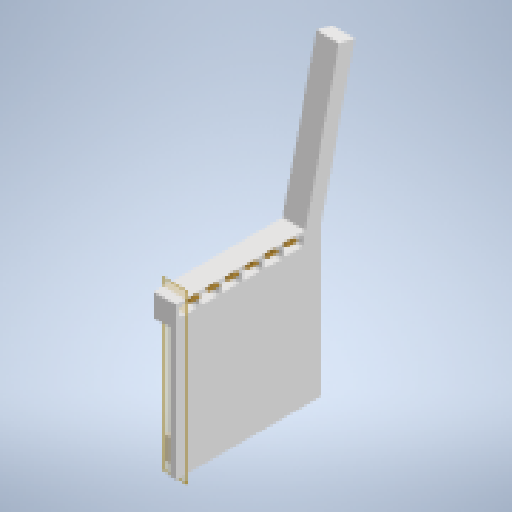
# Autodesk Inventor part: bench-end-peice
Saved by Autodesk Inventor 2023 (Build 270158030, 158C)
## iProperties
Created: 2024-09-09
Part Number: bench-end-peice
Material: Generic
Document SubType Name: Modeling
Designer: Imogen Heard
Density: 1 g/cm^3
Appearance: Default
Author: Imogen Heard
Autodesk Inventor part; units mm, degrees
ref_plane "YZ Plane" through (0, 0, 0) normal (1, 0, 0) x (0, 1, 0)
ref_plane "XZ Plane" through (0, 0, 0) normal (0, 1, 0) x (-1, 0, 0)
ref_plane "XY Plane" through (0, 0, 0) normal (0, 0, 1) x (1, 0, 0)
sketch "Sketch1" plane through (0, 0, 0) normal (1, 0, 0) x (0, 1, 0)
  line L0 (70, 190) -> (0, 190)
  line L1 (0, 190) -> (0, -190)
  line L2 (0, -190) -> (70, -190)
  line L3 (70, -190) -> (70, 190)
  line L4 (29.8496, 82.6594) -> (70, 140)
  line L5 (70, 140) -> (440.1504, -119.1821)
  line L6 (440.1504, -119.1821) -> (400, -176.5227)
  line L7 (400, -176.5227) -> (29.8496, 82.6594)
  line L8 (29.8496, 82.6594) -> (440.1504, -119.1821) construction
  line L9 (70, 140) -> (400, -176.5227) construction
  line L10 (470, 225) -> (400, 225)
  line L11 (400, 225) -> (400, -225)
  line L12 (400, -225) -> (470, -225)
  line L13 (470, -225) -> (470, 225)
  point P0 (0, 0)
  point P1 (35, 190)
  point P2 (435, -225)
  point P3 (400, -91.0685)
  point P4 (70, 54.5458)
  dimension "d0" = 380
  dimension "d1" = 70
  dimension "d2" = 190
  dimension "d3" = 70
  dimension "d4" = 50
  dimension "d5" = 400
  dimension "d6" = 55
  dimension "d7" = -13.4773
  dimension "d8" = 70
  dimension "d9" = 450
  dimension "d10" = 35
  dimension "d11" = 35
  constraints: 28 end point, 6 parallel, 3 perpendicular, 2 horizontal, 2 midpoint, 2 vertical alignment, 1 point on line
  measures "d0" distance between parallel lines of L2 L0
  measures "d1" distance between parallel lines of L3 L1
  measures "d2" distance from line of L0 point (0, 0)
  measures "d3" distance between parallel lines of L7 L5
  measures "d4" vertical distance of point (35, 190) L4.end
  measures "d5" distance from line of L6.end L1
  measures "d6" angle of L3 L7
  measures "d7" distance from line of L2 L6.end
  measures "d8" distance between parallel lines of L11 L13
  measures "d9" distance between parallel lines of L10 L12
  measures "d10" distance from line of point (435, -225) L2
  measures "d11" distance between parallel lines of L10 L0
extrude "Extrusion1" add sketch "Sketch1" along normal blind 70
sketch "Sketch2" plane through (0, 0, 0) normal (-1, 0, 0) x (0, 0, 1)
  line L0 (165, 460) -> (205, 460)
  line L1 (215, 450) -> (215, 440)
  line L2 (205, 430) -> (165, 430)
  line L3 (155, 440) -> (155, 450)
  line L4 (-225, 470) -> (225, 470) projected
  line L5 (225, 470) -> (225, 400) projected
  arc A0 (165, 460) -> (155, 450) centre (165, 450) ccw
  arc A1 (215, 450) -> (205, 460) centre (205, 450) ccw
  arc A2 (205, 430) -> (215, 440) centre (205, 440) ccw
  arc A3 (155, 440) -> (165, 430) centre (165, 440) ccw
  line L6 (100, 460) -> (140, 460)
  line L7 (150, 450) -> (150, 440)
  line L8 (140, 430) -> (100, 430)
  line L9 (90, 440) -> (90, 450)
  arc A4 (100, 460) -> (90, 450) centre (100, 450) ccw
  arc A5 (150, 450) -> (140, 460) centre (140, 450) ccw
  arc A6 (140, 430) -> (150, 440) centre (140, 440) ccw
  arc A7 (90, 440) -> (100, 430) centre (100, 440) ccw
  line L10 (35, 460) -> (75, 460)
  line L11 (85, 450) -> (85, 440)
  line L12 (75, 430) -> (35, 430)
  line L13 (25, 440) -> (25, 450)
  arc A8 (35, 460) -> (25, 450) centre (35, 450) ccw
  arc A9 (85, 450) -> (75, 460) centre (75, 450) ccw
  arc A10 (75, 430) -> (85, 440) centre (75, 440) ccw
  arc A11 (25, 440) -> (35, 430) centre (35, 440) ccw
  line L14 (-30, 460) -> (10, 460)
  line L15 (20, 450) -> (20, 440)
  line L16 (10, 430) -> (-30, 430)
  line L17 (-40, 440) -> (-40, 450)
  arc A12 (-30, 460) -> (-40, 450) centre (-30, 450) ccw
  arc A13 (20, 450) -> (10, 460) centre (10, 450) ccw
  arc A14 (10, 430) -> (20, 440) centre (10, 440) ccw
  arc A15 (-40, 440) -> (-30, 430) centre (-30, 440) ccw
  line L18 (-95, 460) -> (-55, 460)
  line L19 (-45, 450) -> (-45, 440)
  line L20 (-55, 430) -> (-95, 430)
  line L21 (-105, 440) -> (-105, 450)
  arc A16 (-95, 460) -> (-105, 450) centre (-95, 450) ccw
  arc A17 (-45, 450) -> (-55, 460) centre (-55, 450) ccw
  arc A18 (-55, 430) -> (-45, 440) centre (-55, 440) ccw
  arc A19 (-105, 440) -> (-95, 430) centre (-95, 440) ccw
  line L22 (-160, 460) -> (-120, 460)
  line L23 (-110, 450) -> (-110, 440)
  line L24 (-120, 430) -> (-160, 430)
  line L25 (-170, 440) -> (-170, 450)
  arc A20 (-160, 460) -> (-170, 450) centre (-160, 450) ccw
  arc A21 (-110, 450) -> (-120, 460) centre (-120, 450) ccw
  arc A22 (-120, 430) -> (-110, 440) centre (-120, 440) ccw
  arc A23 (-170, 440) -> (-160, 430) centre (-160, 440) ccw
  point P0 (0, 0)
  dimension "d14" = 60
  dimension "d15" = 30
  dimension "d16" = 10
  dimension "d17" = 10
  dimension "d18" = 10
  dimension "d21" = 65
  constraints: 48 end point, 48 point on circle, 24 centre point, 8 tangent, 3 equal radius, 2 horizontal, 2 parallel, 1 perpendicular, 100 other
  measures "d14" distance between parallel lines of L1 L3
  measures "d15" distance between parallel lines of L2 L0
  measures "d16" distance between parallel lines of L4 L0
  measures "d17" distance between parallel lines of L5 L1
  measures "d18" radius of A0
  measures "d21" distance of L0.start L6.start
extrude "Extrusion2" cut sketch "Sketch2" against normal through all
sketch "Sketch3" plane through (70, 0, 0) normal (1, 0, 0) x (0, 0, -1)
  line L0 (223.7185, 458.7524) -> (175, 470)
  line L1 (175, 470) -> (278.8907, 920)
  line L2 (278.8907, 920) -> (327.6092, 908.7524)
  line L3 (327.6092, 908.7524) -> (223.7185, 458.7524)
  line L4 (225, 470) -> (-225, 470) projected
  line L5 (225, 400) -> (225, 470) projected
  line L6 (-225, 470) -> (-225, 400) projected
  point P0 (0, 0)
  point P1 (-225, 435)
  point P2 (225, 435)
  dimension "d28" = 103
  dimension "d29" = 50
  dimension "d30" = 50
  dimension "d31" = 450
  dimension "d32" = 450
  constraints: 8 end point, 2 midpoint, 2 parallel, 1 perpendicular, 1 point on line
  measures "d28" angle of L1 L4
  measures "d29" distance between parallel lines of L3 L1
  measures "d30" distance from line of L5 L0.end
  measures "d31" distance from line of L1.end L4
  measures "d32" distance of point (-225, 435) point (225, 435)
extrude "Extrusion3" add sketch "Sketch3" against normal up to surface (70 mm away)
sketch "Sketch4" plane through (70, 0, 0) normal (1, 0, 0) x (0, 0, -1)
  line L0 (175, 470) -> (-225, 470) projected
  line L1 (-225, 470) -> (-225, 400) projected
  line L2 (-225, 400) -> (91.0685, 400) projected
  line L3 (91.0685, 400) -> (-140, 70) projected
  line L4 (-140, 70) -> (-190, 70) projected
  line L5 (-190, 70) -> (-190, 0) projected
  line L6 (-190, 0) -> (190, 0) projected
  line L7 (190, 0) -> (190, 70) projected
  line L8 (190, 70) -> (-54.5458, 70) projected
  line L9 (-54.5458, 70) -> (176.5227, 400) projected
  line L10 (176.5227, 400) -> (225, 400) projected
  line L11 (225, 400) -> (225, 464.3032) projected
  line L12 (225, 464.3032) -> (327.6092, 908.7524) projected
  line L13 (327.6092, 908.7524) -> (278.8907, 920) projected
  line L14 (278.8907, 920) -> (175, 470) projected
  arc A0 (-20, 440) -> (-10, 430) centre (-10, 440) ccw projected
  line L15 (-20, 440) -> (-20, 450) projected
  arc A1 (-10, 460) -> (-20, 450) centre (-10, 450) ccw projected
  line L16 (-10, 460) -> (30, 460) projected
  arc A2 (40, 450) -> (30, 460) centre (30, 450) ccw projected
  line L17 (40, 450) -> (40, 440) projected
  arc A3 (30, 430) -> (40, 440) centre (30, 440) ccw projected
  line L18 (30, 430) -> (-10, 430) projected
  arc A4 (-215, 440) -> (-205, 430) centre (-205, 440) ccw projected
  line L19 (-215, 440) -> (-215, 450) projected
  arc A5 (-205, 460) -> (-215, 450) centre (-205, 450) ccw projected
  line L20 (-205, 460) -> (-165, 460) projected
  arc A6 (-155, 450) -> (-165, 460) centre (-165, 450) ccw projected
  line L21 (-155, 450) -> (-155, 440) projected
  arc A7 (-165, 430) -> (-155, 440) centre (-165, 440) ccw projected
  line L22 (-165, 430) -> (-205, 430) projected
  arc A8 (45, 440) -> (55, 430) centre (55, 440) ccw projected
  line L23 (45, 440) -> (45, 450) projected
  arc A9 (55, 460) -> (45, 450) centre (55, 450) ccw projected
  line L24 (55, 460) -> (95, 460) projected
  arc A10 (105, 450) -> (95, 460) centre (95, 450) ccw projected
  line L25 (105, 450) -> (105, 440) projected
  arc A11 (95, 430) -> (105, 440) centre (95, 440) ccw projected
  line L26 (95, 430) -> (55, 430) projected
  arc A12 (-85, 440) -> (-75, 430) centre (-75, 440) ccw projected
  line L27 (-85, 440) -> (-85, 450) projected
  arc A13 (-75, 460) -> (-85, 450) centre (-75, 450) ccw projected
  line L28 (-75, 460) -> (-35, 460) projected
  arc A14 (-25, 450) -> (-35, 460) centre (-35, 450) ccw projected
  line L29 (-25, 450) -> (-25, 440) projected
  arc A15 (-35, 430) -> (-25, 440) centre (-35, 440) ccw projected
  line L30 (-35, 430) -> (-75, 430) projected
  arc A16 (-150, 440) -> (-140, 430) centre (-140, 440) ccw projected
  line L31 (-150, 440) -> (-150, 450) projected
  arc A17 (-140, 460) -> (-150, 450) centre (-140, 450) ccw projected
  line L32 (-140, 460) -> (-100, 460) projected
  arc A18 (-90, 450) -> (-100, 460) centre (-100, 450) ccw projected
  line L33 (-90, 450) -> (-90, 440) projected
  arc A19 (-100, 430) -> (-90, 440) centre (-100, 440) ccw projected
  line L34 (-100, 430) -> (-140, 430) projected
  arc A20 (110, 440) -> (120, 430) centre (120, 440) ccw projected
  line L35 (110, 440) -> (110, 450) projected
  arc A21 (120, 460) -> (110, 450) centre (120, 450) ccw projected
  line L36 (120, 460) -> (160, 460) projected
  arc A22 (170, 450) -> (160, 460) centre (160, 450) ccw projected
  line L37 (170, 450) -> (170, 440) projected
  arc A23 (160, 430) -> (170, 440) centre (160, 440) ccw projected
  line L38 (160, 430) -> (120, 430) projected
  line L39 (-225, 400) -> (91.0685, 400) projected
  line L40 (-225, 400) -> (225, 400)
  line L41 (225, 400) -> (225, 0)
  line L42 (225, 0) -> (-225, 0)
  line L43 (-225, 0) -> (-225, 400)
  point P0 (0, 0)
  point P1 (190, 0)
  constraints: 8 end point, 2 coincident, 2 parallel, 1 horizontal, 1 perpendicular
extrude "Extrusion4" add sketch "Sketch4" against normal blind 20 contours L2 L3 L4 L5 L42 L43 | L10 L41 L42 L7 L8 L9
ref_plane "Work Plane1" through (0, 400, 195) normal (0, 0, 1) x (1, 0, 0)
sketch "Sketch6" plane through (0, 400, 195) normal (0, 0, 1) x (1, 0, 0)
  line L0 (70, 70) -> (70, -400) projected
  line L1 (79, 64) -> (79, 60) projected
  arc A0 (83, 65) -> (79, 60) centre (88.3977, 56.5819) ccw projected
  arc A1 (83, 65) -> (79, 60) centre (88.3977, 56.5819) ccw projected
  line L2 (70, -400) -> (70, 64.3032) projected
  line L3 (70, 64.3032) -> (70, 508.7524) projected
  line L4 (70.101, 64) -> (79, 64) projected
  arc A2 (70.101, 64) -> (75.101, 70) centre (65.5288, 72.8935) ccw projected
  arc A3 (83, 65) -> (75.101, 70) centre (80, 69) ccw projected
  arc A4 (83, 65) -> (79, 60) centre (88.3977, 56.5819) ccw projected
  line L5 (79, 64) -> (79, 60) projected
  circle A5 centre (80, 69) radius 3.5 projected
  arc A6 (80, 64) -> (70, 60.5) centre (79.281, 50.0185) ccw
  line L6 (79, 64) -> (79, 34) projected
  circle A7 centre (80, 69) radius 5
  line L7 (70, 69.5) -> (75.0251, 69.5)
  point P0 (0, -400)
  point P1 (82.5951, 64.7262)
  point P2 (83, 65)
  point P3 (85, 69)
  point P4 (70, 69.5)
  point P5 (70, 60.5)
  point P6 (77.4412, 63.8971)
  point P7 (79.6218, 64.0143)
  point P8 (77, 65)
  point P9 (75.069, 69.8276)
  point P10 (75.101, 70)
  point P11 (77.0437, 63.8385)
  point P12 (78.9215, 64.0139)
  point P13 (76.8404, 64.3811)
  point P14 (70, 65.5882)
  point P15 (83, 65)
  point P16 (82.5951, 64.7262)
  point P17 (83, 65)
  point P18 (82.5951, 64.7262)
  point P19 (60.176, 67.3219)
  point P20 (70, 50.8991)
  dimension "d40" = 0.5
  dimension "d41" = 9
  dimension "d42" = 14
  dimension "d43" = 8.5
  constraints: 3 point on circle, 2 end point, 2 point on line, 1 centre point, 1 perpendicular, 1 vertical alignment, 6 other
  measures "d41" distance of L7.start A6.end
  measures "d42" radius of A6
  measures "d43" vertical distance of A3.centre A6.end
extrude "Extrusion5" add sketch "Sketch6" against normal blind 30 separate body contours L7 A2 L4 A6 L0 | L7 A7 A6 L4 A2 | A3 A0 A7 A6 | A6 A7
pattern_linear "Rectangular Pattern1" count 6 spacing 60 along (0, 0, -1) bodies 2
sketch "Sketch7" plane through (0, 0, 0) normal (-1, 0, 0) x (0, 0, 1)
  circle A0 centre (-206.763, 492) radius 12.5
  line L0 (-327.6092, 908.7524) -> (-225, 464.3032) projected
  line L1 (-175, 470) -> (225, 470) projected
  point P0 (0, 0)
  dimension "d49" = 25
  dimension "d50" = 24
  dimension "d51" = 22
  constraints: 1 centre point
  measures "d49" diameter of A0
  measures "d50" distance from line of L0 A0.centre
  measures "d51" distance from line of L1 A0.centre
extrude "Extrusion6" add sketch "Sketch7" along normal blind 30 separate body
fillet "Fillet1" radius 4 1 edges at (-30, 492, -219.263)
sketch "Sketch8" plane through (0, 0, 0) normal (-1, 0, 0) x (0, 0, 1)
  line L0 (-305.4994, 924.1199) -> (-280.7548, 816.9392) construction
  line L1 (-327.6092, 908.7524) -> (-278.8907, 920) projected
  line L2 (-292.8326, 927.0443) -> (-268.088, 819.8636)
  line L3 (-293.4216, 814.0149) -> (-318.1663, 921.1956)
  arc A0 (-292.8326, 927.0443) -> (-318.1663, 921.1956) centre (-305.4994, 924.1199) ccw
  arc A1 (-293.4216, 814.0149) -> (-268.088, 819.8636) centre (-280.7548, 816.9392) ccw
  line L4 (-327.6092, 908.7524) -> (-225, 464.3032) projected
  line L5 (-175, 470) -> (-278.8907, 920) projected
  point P0 (0, 0)
  point P1 (-293.1271, 870.5296)
  point P2 (-290.5831, 917.3006)
  point P3 (-315.9167, 911.4519)
  dimension "d55" = 26
  dimension "d56" = 12
  dimension "d57" = 12
  dimension "d58" = 100
  dimension "d59" = 10
  constraints: 8 end point, 4 point on circle, 4 tangent, 2 centre point, 1 midpoint, 1 parallel, 1 perpendicular
  measures "d55" distance between parallel lines of L3 L2
  measures "d56" distance between parallel lines of L3 L4
  measures "d57" distance between parallel lines of L5 L2
  measures "d58" distance from line of L1 L0.end
  measures "d59" distance from line of L1 L0.start
extrude "Extrusion7" cut sketch "Sketch8" against normal blind 30 contours L1 L2 A1 L3 bodies 1
equation "\"d2\" = 0.5 * d0"
equation "\"d10\" = -0.5 * d0 + 0.5 * d9"
body "Solid1"
